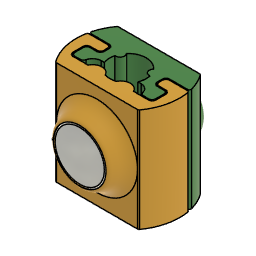
cableMag v10 (Autodesk Fusion 360 design; units mm, degrees)
Autodesk Fusion 360 part; units mm, degrees
note: some values were not read from the file. Set by a fixed rule: which face or edge a step refers to.
sketch "Sketch1" plane through (0, 0, 0) normal (0, 0, 1) x (1, 0, 0)
  circle A0 centre (0, 0) radius 2.1
  circle A1 centre (0, 0) radius 6
  line L0 (0, 7.6694) -> (0, -7.0852)
  line L1 (-3.2, 7.6694) -> (-3.2, -7.0852)
  line L2 (-4.8, 7.6694) -> (-4.8, -7.0852)
  line L3 (4.8, 7.6694) -> (4.8, -7.0852)
  line L4 (3.2, 7.6694) -> (3.2, -7.0852)
  line L5 (-7.6365, 0) -> (7.8861, 0)
  line L6 (-7.6365, -0.8) -> (7.8861, -0.8)
  line L7 (-7.6365, -2) -> (7.8861, -2)
  line L8 (-7.6365, -3.6) -> (7.8861, -3.6)
  line L9 (-7.6365, 1.2) -> (7.8861, 1.2)
  line L10 (-4.8, -3.6) -> (4.8, -3.6)
  line L11 (-5.6569, -2) -> (-0.6403, -2)
  line L12 (0.6403, -2) -> (5.6569, -2)
  line L13 (-2.1, 0) -> (-3.2, 0)
  line L14 (-3.2, -0.8) -> (-4.8, -0.8)
  line L15 (-4.8, -0.8) -> (-4.8, -2)
  line L16 (-3.2, 0) -> (-3.2, -0.8)
  line L17 (2.1, 0) -> (3.2, 0)
  line L18 (3.2, -0.8) -> (3.2, 0)
  line L19 (3.2, -0.8) -> (4.8, -0.8)
  line L20 (4.8, -0.8) -> (4.8, -2)
  line L21 (-7.6365, 3.6) -> (7.8861, 3.6)
  line L22 (-5.8788, 1.2) -> (-1.7234, 1.2)
  line L23 (1.7234, 1.2) -> (5.8788, 1.2)
  dimension "d2" = 4.2
  dimension "d7" = 12
  dimension "d9" = 3.2
  dimension "d10" = 4.8
  dimension "d11" = 0.8
  dimension "d12" = 2
  dimension "d13" = 3.6
  dimension "d14" = -1.2
  dimension "d15" = -3.6
  constraint coincident A0.centre A1.centre
  constraint symmetric L0 L1.start L4.start
  constraint symmetric L0 L1.end L4.end
  constraint symmetric L0 L2.start L3.start
  constraint symmetric L0 L2.end L3.end
  constraint perpendicular L3 L5
  constraint coincident A1 L10.start
  constraint coincident L8 L10.start
  constraint coincident A1 L10.end
  constraint coincident L8 L10.end
  constraint coincident A1 L11.start
  constraint coincident L7 L11.start
  constraint coincident A0 L11.end
  constraint coincident L7 L11.end
  constraint coincident A0 L12.start
  constraint coincident L7 L12.start
  constraint coincident A1 L12.end
  constraint coincident L7 L12.end
  constraint coincident A0 L13.start
  constraint coincident L5 L13.start
  constraint coincident L5 L13.end
  constraint coincident L1 L13.end
  constraint perpendicular L1 L13
  constraint coincident L1 L14.start
  constraint coincident L6 L14.start
  constraint coincident L6 L14.end
  constraint coincident L2 L14.end
  constraint coincident L2 L15.end
  constraint coincident L7 L15.end
  constraint coincident A0 L17.start
  constraint coincident L5 L17.start
  constraint coincident L4 L17.end
  constraint coincident L5 L17.end
  constraint perpendicular L4 L17
  constraint coincident L4 L18.start
  constraint coincident L6 L18.start
  constraint coincident L6 L19.end
  constraint coincident L3 L19.end
  constraint vertical L20
  constraint coincident L7 L20.end
  constraint coincident L9 L22.start
  constraint coincident A1 L22.start
  constraint coincident L9 L22.end
  constraint coincident A0 L22.end
  constraint coincident A0 L23.start
  constraint coincident L9 L23.start
  constraint coincident A1 L23.end
  constraint coincident L9 L23.end
  constraint perpendicular L4 L23
  measures "d2" diameter of A0
  measures "d7" diameter of A1
extrude "Extrude1" add sketch "Sketch1" along normal blind 12 contours L3 L4 L5 L9 L23 | A0 L0 L4 L7 L8 L10 L12 | A1 L3 L5 L6 | A1 L3 L5 L9 L23 | A0 L0 L1 L7 L8 L10 L11 | L3 L4 L7 L8 L10 L12 | A1 L3 L6 L7 L12 L20 | L1 L2 L5 L9 L22 | A1 L3 L7 L12 | A1 L2 L5 L9 L22 | A1 L2 L5 L6 | L1 L2 L7 L8 L10 L11 | A1 L2 L6 L7 L11 L15 | A1 L2 L7 L11 makes body 1
extrude "Extrude2" add sketch "Sketch1" along normal blind 12 separate body contours A0 L4 L5 L6 L17 L18 | A0 L4 L5 L9 L17 L23 | A0 L0 L4 L9 L21 L23 | L3 L4 L5 L6 L18 L19 | A0 L0 L1 L9 L21 L22 | L3 L4 L9 L21 L23 | L3 L4 L6 L7 L12 L19 L20 | A0 L1 L5 L9 L13 L22 | A0 L1 L5 L6 L13 L16 | A1 L3 L9 L23 | L1 L2 L5 L6 L14 L16 | L1 L2 L9 L21 L22 | L1 L2 L6 L7 L11 L14 L15 | A1 L2 L9 L22 makes body 2
copy_body "Body->Comp1" bodies 1 removing the originals makes body 3 in component "bottom"
copy_body "Body->Comp2" bodies 2 removing the originals makes body 4 in component "top"
move_face "OffsetFaces1" offset -0.12 16 faces at (3.7333, 1.2, 4) (5.1596, 1.2, 4) (3.2, 0.8, 4) (3.7333, 0, 4) (4.8, -1.2, 4) (4.8, -0.2667, 4) (3.7333, -2, 4) (3.2, -1.2, 4) (-3.2, -1.2, 4) (-4.2667, -2, 4) (-4.8, -0.2667, 4) (-4.8, -1.2, 4) (-4.2667, 0, 4) (-3.2, 0.8, 4) (-5.5192, 1.2, 4) (-4.2667, 1.2, 4) on bodies 4 in component "top"
fillet "Fillet1" radius 0.4 2 edges at (4.68, -0.12, 6) (-4.68, -0.12, 6) on bodies 4 in component "top"
fillet "Fillet2" radius 0.4 2 edges at (4.68, -1.88, 6) (-4.68, -1.88, 6) on bodies 4 in component "top"
fillet "Fillet1'" radius 0.4 4 edges at (4.8, -2, 6) (-4.8, -2, 6) (-4.8, 0, 6) (4.8, 0, 6) on bodies 3 in component "bottom"
fillet "Fillet2'" radius 0.4 4 edges at (3.2, 1.2, 6) (3.2, 0, 6) (-3.2, 1.2, 6) (-3.2, 0, 6) on bodies 3 in component "bottom"
fillet "Fillet4" radius 0.4 4 edges at (3.08, 1.32, 6) (3.08, -0.12, 6) (-3.08, 1.32, 6) (-3.08, -0.12, 6) on bodies 4 in component "top"
fillet "Fillet5" radius 1 2 edges at (3.32, -0.8, 6) (-3.32, -0.8, 6) on bodies 4 in component "top"
fillet "Fillet6" radius 0.4 2 edges at (3.32, -1.88, 6) (-3.32, -1.88, 6) on bodies 4 in component "top"
fillet "Fillet3" radius 0.2 4 edges at (-4.8, -3.6, 6) (4.8, -3.6, 6) (5.8788, 1.2, 6) (-5.8788, 1.2, 6) on bodies 3 in component "bottom"
fillet "Fillet7" radius 0.2 4 edges at (4.8, 3.6, 6) (-4.8, 3.6, 6) (5.853, 1.32, 6) (-5.853, 1.32, 6) on bodies 4 in component "top"
sketch "Sketch2" plane through (0, 3.6, 0) normal (0, 1, 0) x (-1, 0, 0)
  line L0 (4.6989, 0) -> (4.6989, 12)
  line L1 (4.6989, 12) -> (-4.6989, 12)
  line L2 (-4.6989, 12) -> (-4.6989, 0)
  line L3 (-4.6989, 0) -> (4.6989, 0)
  line L4 (0, -1.5126) -> (0, 13.7885) construction
  line L5 (6.4261, 6) -> (-15.824, 6) construction
  circle A0 centre (0, 6) radius 3.05
  dimension "d44" = 6.1
  constraint perpendicular L3 L4
  constraint perpendicular L2 L5
  constraint midpoint L2 L5
  constraint coincident L4 A0.centre
  constraint coincident L5 A0.centre
  measures "d44" diameter of A0
extrude "Extrude3" add sketch "Sketch2" along normal blind 2 separate body contours A0 makes body 5
ref_plane "WorkPlane1" through (0, 0, 6) normal (0, 0, 1) x (1, 0, 0)
copy_body "Body->Comp3" bodies 5 removing the originals makes body 6 in component "magnet"
sketch "Sketch3" plane through (0, 0, 6) normal (0, 0, 1) x (1, 0, 0)
  line L0 (3.05, 5.6) -> (-3.05, 5.6)
  line L1 (3.05, 3.6) -> (-3.05, 3.6)
  arc A0 (-5.7903, 1.5724) -> (-5.5973, 1.32) centre (-5.5973, 1.52) ccw
  arc A1 (-4.861, 3.5172) -> (-5.7903, 1.5724) centre (0, 0) ccw
  arc A2 (-4.6989, 3.6) -> (-4.861, 3.5172) centre (-4.6989, 3.4) ccw
  line L2 (-4.6989, 3.6) -> (4.6989, 3.6)
  arc A3 (4.861, 3.5172) -> (4.6989, 3.6) centre (4.6989, 3.4) ccw
  arc A4 (5.7903, 1.5724) -> (4.861, 3.5172) centre (0, 0) ccw
  arc A5 (5.5973, 1.32) -> (5.7903, 1.5724) centre (5.5973, 1.52) ccw
  line L3 (5.5973, 1.32) -> (3.48, 1.32)
  arc A6 (3.48, 1.32) -> (3.08, 0.92) centre (3.48, 0.92) ccw
  line L4 (3.08, 0.92) -> (3.08, 0.28)
  arc A7 (3.08, 0.28) -> (3.48, -0.12) centre (3.48, 0.28) ccw
  line L5 (3.48, -0.12) -> (4.28, -0.12)
  arc A8 (4.68, -0.52) -> (4.28, -0.12) centre (4.28, -0.52) ccw
  line L6 (4.68, -0.52) -> (4.68, -1.48)
  arc A9 (4.28, -1.88) -> (4.68, -1.48) centre (4.28, -1.48) ccw
  line L7 (4.28, -1.88) -> (3.6829, -1.88)
  arc A10 (3.2935, -1.5714) -> (3.6829, -1.88) centre (3.6829, -1.48) ccw
  arc A11 (3.2935, -1.5714) -> (2.32, -0.8) centre (2.32, -1.8) ccw
  line L8 (2.32, -0.8) -> (1.9416, -0.8)
  arc A12 (1.9416, -0.8) -> (-1.9416, -0.8) centre (0, 0) ccw
  line L9 (-1.9416, -0.8) -> (-2.32, -0.8)
  arc A13 (-2.32, -0.8) -> (-3.2935, -1.5714) centre (-2.32, -1.8) ccw
  arc A14 (-3.6829, -1.88) -> (-3.2935, -1.5714) centre (-3.6829, -1.48) ccw
  line L10 (-3.6829, -1.88) -> (-4.28, -1.88)
  arc A15 (-4.68, -1.48) -> (-4.28, -1.88) centre (-4.28, -1.48) ccw
  line L11 (-4.68, -1.48) -> (-4.68, -0.52)
  arc A16 (-4.28, -0.12) -> (-4.68, -0.52) centre (-4.28, -0.52) ccw
  line L12 (-4.28, -0.12) -> (-3.48, -0.12)
  arc A17 (-3.48, -0.12) -> (-3.08, 0.28) centre (-3.48, 0.28) ccw
  line L13 (-3.08, 0.28) -> (-3.08, 0.92)
  arc A18 (-3.08, 0.92) -> (-3.48, 1.32) centre (-3.48, 0.92) ccw
  line L14 (-3.48, 1.32) -> (-5.5973, 1.32)
  arc A19 (-5.7131, 1.2) -> (-5.9101, 1.0345) centre (-5.7131, 1) ccw
  line L15 (-5.7131, 1.2) -> (-3.6, 1.2)
  arc A20 (-3.2, 0.8) -> (-3.6, 1.2) centre (-3.6, 0.8) ccw
  line L16 (-3.2, 0.8) -> (-3.2, 0.4)
  arc A21 (-3.6, 0) -> (-3.2, 0.4) centre (-3.6, 0.4) ccw
  line L17 (-3.6, 0) -> (-4.4, 0)
  arc A22 (-4.4, 0) -> (-4.8, -0.4) centre (-4.4, -0.4) ccw
  line L18 (-4.8, -0.4) -> (-4.8, -1.6)
  arc A23 (-4.8, -1.6) -> (-4.4, -2) centre (-4.4, -1.6) ccw
  line L19 (-4.4, -2) -> (-0.6403, -2)
  arc A24 (-0.6403, -2) -> (0.6403, -2) centre (0, 0) ccw
  line L20 (0.6403, -2) -> (4.4, -2)
  arc A25 (4.4, -2) -> (4.8, -1.6) centre (4.4, -1.6) ccw
  line L21 (4.8, -1.6) -> (4.8, -0.4)
  arc A26 (4.8, -0.4) -> (4.4, 0) centre (4.4, -0.4) ccw
  line L22 (4.4, 0) -> (3.6, 0)
  arc A27 (3.2, 0.4) -> (3.6, 0) centre (3.6, 0.4) ccw
  line L23 (3.2, 0.4) -> (3.2, 0.8)
  arc A28 (3.6, 1.2) -> (3.2, 0.8) centre (3.6, 0.8) ccw
  line L24 (3.6, 1.2) -> (5.7131, 1.2)
  arc A29 (5.9101, 1.0345) -> (5.7131, 1.2) centre (5.7131, 1) ccw
  arc A30 (4.861, -3.5172) -> (5.9101, 1.0345) centre (0, 0) ccw
  arc A31 (4.6989, -3.6) -> (4.861, -3.5172) centre (4.6989, -3.4) ccw
  line L25 (4.6989, -3.6) -> (-4.6989, -3.6)
  arc A32 (-4.861, -3.5172) -> (-4.6989, -3.6) centre (-4.6989, -3.4) ccw
  arc A33 (-5.9101, 1.0345) -> (-4.861, -3.5172) centre (0, 0) ccw
  line L26 (-3.05, 5.6) -> (-3.05, 3.6)
  spline S0 degree 5 poles (-4.6989, 3.6) (-4.6667, 3.6196) (-4.603, 3.6598) (-4.5103, 3.7233) (-4.3921, 3.8143) (-4.2537, 3.9389) (-4.125, 4.0745) (-4.006, 4.2213) (-3.8969, 4.3787) (-3.7972, 4.5459) (-3.7062, 4.7211) (-3.6222, 4.9009) (-3.5427, 5.0801) (-3.4644, 5.251) (-3.3821, 5.4024) (-3.29, 5.5214) (-3.204, 5.5806) (-3.1307, 5.6004) (-3.0776, 5.602) (-3.05, 5.6) knots 0 0 0 0 0 0 0.066667 0.133333 0.2 0.266667 0.333333 0.4 0.466667 0.533333 0.6 0.666667 0.733333 0.8 0.866667 0.933333 1 1 1 1 1 1
  line L27 (-3.2911, 5.6178) -> (-2.8089, 5.5822)
  line L28 (-4.1639, 4.0124) -> (-3.8238, 4.4748)
  line L29 (-7.2966, 0) -> (7.3737, 0) construction
  spline S1 degree 5 poles (-4.6989, -3.6) (-4.6667, -3.6196) (-4.603, -3.6598) (-4.5103, -3.7233) (-4.3921, -3.8143) (-4.2537, -3.9389) (-4.125, -4.0745) (-4.006, -4.2213) (-3.8969, -4.3787) (-3.7972, -4.5459) (-3.7062, -4.7211) (-3.6222, -4.9009) (-3.5427, -5.0801) (-3.4644, -5.251) (-3.3821, -5.4024) (-3.29, -5.5214) (-3.204, -5.5806) (-3.1307, -5.6004) (-3.0776, -5.602) (-3.05, -5.6) knots 0 0 0 0 0 0 0.066667 0.133333 0.2 0.266667 0.333333 0.4 0.466667 0.533333 0.6 0.666667 0.733333 0.8 0.866667 0.933333 1 1 1 1 1 1
  line L30 (-4.947, 3.4494) -> (-4.4509, 3.7506)
  line L31 (-4.947, -3.4494) -> (-4.4509, -3.7506)
  line L32 (-4.1639, -4.0124) -> (-3.8238, -4.4748)
  line L33 (-3.2911, -5.6178) -> (-2.8089, -5.5822)
  line L34 (-3.05, -5.6) -> (-3.05, -3.6)
  point P0 (-3.9939, 4.2436)
  point P1 (-3.5155, 5.1379)
  point P2 (-3.9939, -4.2436)
  point P3 (-3.5155, -5.1379)
  constraint coincident L0.end L26.start
  constraint coincident L1.end L26.end
  constraint coincident A2.start L2.start
  constraint midpoint L0.end L27
  constraint midpoint P0 L28
  constraint parallel L22 L29
  constraint midpoint A2.start L30
  constraint symmetric L0.end L29 S1.end
  constraint symmetric L1.end L29 L34.end
  constraint symmetric A2.start L29 L25.end
  constraint symmetric P0 L29 P2
  constraint symmetric P1 L29 P3
  constraint symmetric L27.start L29 L33.start
  constraint symmetric L27.end L29 L33.end
  constraint symmetric L28.start L29 L32.start
  constraint symmetric L28.end L29 L32.end
  constraint symmetric L29 L30.start L31.start
  constraint symmetric L29 L30.end L31.end
revolve "Revolve1" add sketch "Sketch3" angle 360 about axis through (0, 2.6, 6) along (0, 1, 0) contours L2 L26 S0 bodies 4 in component "top"
revolve "Revolve1'" add sketch "Sketch3" angle 360 about axis through (0, 2.6, 6) along (0, 1, 0) contours L25 S1 L34 bodies 3 in component "bottom"
sketch "Sketch4" plane through (0, 0, 12) normal (0, 0, 1) x (-1, 0, 0)
  arc A0 (5.7131, -1.2) -> (5.9101, -1.0345) centre (5.7131, -1) ccw
  arc A1 (5.9101, -1.0345) -> (4.861, 3.5172) centre (0, 0) ccw
  arc A2 (4.861, 3.5172) -> (4.6989, 3.6) centre (4.6989, 3.4) ccw
  line L0 (4.6989, 3.6) -> (-4.6989, 3.6)
  arc A3 (-4.6989, 3.6) -> (-4.861, 3.5172) centre (-4.6989, 3.4) ccw
  arc A4 (-4.861, 3.5172) -> (-5.9101, -1.0345) centre (0, 0) ccw
  arc A5 (-5.9101, -1.0345) -> (-5.7131, -1.2) centre (-5.7131, -1) ccw
  line L1 (-5.7131, -1.2) -> (-3.6, -1.2)
  arc A6 (-3.6, -1.2) -> (-3.2, -0.8) centre (-3.6, -0.8) ccw
  line L2 (-3.2, -0.8) -> (-3.2, -0.4)
  arc A7 (-3.2, -0.4) -> (-3.6, 0) centre (-3.6, -0.4) ccw
  line L3 (-3.6, 0) -> (-4.4, 0)
  arc A8 (-4.8, 0.4) -> (-4.4, 0) centre (-4.4, 0.4) ccw
  line L4 (-4.8, 0.4) -> (-4.8, 1.6)
  arc A9 (-4.4, 2) -> (-4.8, 1.6) centre (-4.4, 1.6) ccw
  line L5 (-4.4, 2) -> (-0.6403, 2)
  arc A10 (0.6403, 2) -> (-0.6403, 2) centre (0, 0) ccw
  line L6 (0.6403, 2) -> (4.4, 2)
  arc A11 (4.8, 1.6) -> (4.4, 2) centre (4.4, 1.6) ccw
  line L7 (4.8, 1.6) -> (4.8, 0.4)
  arc A12 (4.4, 0) -> (4.8, 0.4) centre (4.4, 0.4) ccw
  line L8 (4.4, 0) -> (3.6, 0)
  arc A13 (3.6, 0) -> (3.2, -0.4) centre (3.6, -0.4) ccw
  line L9 (3.2, -0.4) -> (3.2, -0.8)
  arc A14 (3.2, -0.8) -> (3.6, -1.2) centre (3.6, -0.8) ccw
  line L10 (3.6, -1.2) -> (5.7131, -1.2)
  line L11 (0, 0) -> (0, 6.5726) construction
  arc A15 (0.6403, 2) -> (2.6403, 2) centre (1.6403, 2.4718) ccw
  arc A16 (-2.6403, 2) -> (-0.6403, 2) centre (-1.6403, 2.4718) ccw
  arc A17 (5.7903, -1.5724) -> (5.5973, -1.32) centre (5.5973, -1.52) ccw
  line L12 (5.5973, -1.32) -> (3.48, -1.32)
  arc A18 (3.08, -0.92) -> (3.48, -1.32) centre (3.48, -0.92) ccw
  line L13 (3.08, -0.92) -> (3.08, -0.28)
  arc A19 (3.48, 0.12) -> (3.08, -0.28) centre (3.48, -0.28) ccw
  line L14 (3.48, 0.12) -> (4.28, 0.12)
  arc A20 (4.28, 0.12) -> (4.68, 0.52) centre (4.28, 0.52) ccw
  line L15 (4.68, 0.52) -> (4.68, 1.48)
  arc A21 (4.68, 1.48) -> (4.28, 1.88) centre (4.28, 1.48) ccw
  line L16 (4.28, 1.88) -> (3.6829, 1.88)
  arc A22 (3.6829, 1.88) -> (3.2935, 1.5714) centre (3.6829, 1.48) ccw
  arc A23 (2.32, 0.8) -> (3.2935, 1.5714) centre (2.32, 1.8) ccw
  line L17 (2.32, 0.8) -> (1.9416, 0.8)
  arc A24 (-1.9416, 0.8) -> (1.9416, 0.8) centre (0, 0) ccw
  line L18 (-1.9416, 0.8) -> (-2.32, 0.8)
  arc A25 (-3.2935, 1.5714) -> (-2.32, 0.8) centre (-2.32, 1.8) ccw
  arc A26 (-3.2935, 1.5714) -> (-3.6829, 1.88) centre (-3.6829, 1.48) ccw
  line L19 (-3.6829, 1.88) -> (-4.28, 1.88)
  arc A27 (-4.28, 1.88) -> (-4.68, 1.48) centre (-4.28, 1.48) ccw
  line L20 (-4.68, 1.48) -> (-4.68, 0.52)
  arc A28 (-4.68, 0.52) -> (-4.28, 0.12) centre (-4.28, 0.52) ccw
  line L21 (-4.28, 0.12) -> (-3.48, 0.12)
  arc A29 (-3.08, -0.28) -> (-3.48, 0.12) centre (-3.48, -0.28) ccw
  line L22 (-3.08, -0.28) -> (-3.08, -0.92)
  arc A30 (-3.48, -1.32) -> (-3.08, -0.92) centre (-3.48, -0.92) ccw
  line L23 (-3.48, -1.32) -> (-5.5973, -1.32)
  arc A31 (-5.5973, -1.32) -> (-5.7903, -1.5724) centre (-5.5973, -1.52) ccw
  arc A32 (-5.7903, -1.5724) -> (-4.861, -3.5172) centre (0, 0) ccw
  arc A33 (-4.861, -3.5172) -> (-4.6989, -3.6) centre (-4.6989, -3.4) ccw
  line L24 (-4.6989, -3.6) -> (4.6989, -3.6)
  arc A34 (4.6989, -3.6) -> (4.861, -3.5172) centre (4.6989, -3.4) ccw
  arc A35 (4.861, -3.5172) -> (5.7903, -1.5724) centre (0, 0) ccw
  arc A36 (2.0374, -0.5088) -> (1.5711, -1.3934) centre (1.9442, -1.0249) ccw
  arc A37 (-1.5711, -1.3934) -> (-2.0374, -0.5088) centre (-1.9442, -1.0249) ccw
  dimension "d50" = 2
  dimension "d53" = 1
  constraint coincident A1.centre A4.centre
  constraint vertical L11
  constraint coincident L6 A15.end
  constraint coincident A10.start L6.start
  constraint symmetric L11 A10.start L5.end
  constraint symmetric L11 A15.end A16.start
  constraint symmetric L11 A15 A16
  constraint coincident A24 A36.end
  constraint coincident A24 A36.start
  constraint symmetric L11 A36.start A37.end
  constraint symmetric L11 A36.end A37.start
  constraint symmetric L11 A36 A37
  measures "d50" distance of A10.start A15.end
  measures "d53" distance of A36.start A36.end
extrude "Extrude1'" add sketch "Sketch4" against normal up to surface (12 mm away) contours L6 A15 | L5 A16 | A24 A36 | A24 A37 bodies 3 makes body 7 at (-1.4198, 1.0175, 4) makes body 8 at (1.4921, 1.2906, 4) in component "bottom"
combine "Combine1" operation add target body 8 tool bodies 7 4 in component "bottom"
fillet "Fillet1''" radius 0.2 2 edges at (2.8436, 5.6, 4.8971) (2.8436, 3.6, 4.8971) on bodies 6 in component "magnet"
copy_body "CopyPasteBodies1" bodies 6 makes body 9 in component "magnet"
move_body "Move1" bodies 9 to x (1, 0, 0) y (0, 1, 0) z (0, 0, 1) at (0, -9.2, 0) in component "magnet"
component "bottom" placed x (1, 0, 0) y (0, 1, 0) z (0, 0, 1) at (0, 0, 0)
component "top" placed x (1, 0, 0) y (0, 1, 0) z (0, 0, 1) at (0, 0, 0)
component "magnet" placed x (1, 0, 0) y (0, 1, 0) z (0, 0, 1) at (0, 0, 0)
equation "cableDia = 4.2 mm"
equation "d2 = cableDia"
equation "shellWid = 10 mm"
equation "shellDep = 8 mm"
equation "d7 = shellDia"
equation "shellDia = 12 mm"
equation "faceOff = 0.12 mm"
equation "d21 = -faceOff"
equation "slideFilet = 0.8 mm"
equation "magDia = 6.1 mm"
equation "d44 = magDia"
named bodies: "magnet", "magnet (1)"
